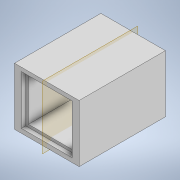
# Autodesk Inventor part: Part2
Saved by Autodesk Inventor 2022.6 (Build 266554010, 554A)
## iProperties
Created: 2025-03-19
Part Number: Part2
Material: Generic
Document SubType Name: Modeling
Designer: khinm
Density: 1 g/cm^3
Appearance: Default
Author: khinm
Autodesk Inventor part; units mm, degrees
ref_plane "XZ Plane" through (0, 0, 0) normal (0, 1, 0) x (-1, 0, 0)
ref_plane "XY Plane" through (0, 0, 0) normal (0, 0, 1) x (1, 0, 0)
sketch "Sketch1" plane through (0, 0, 0) normal (0, 0, 1) x (1, 0, 0)
  line L0 (-9.4982, 16.8551) -> (9.4982, 16.8551)
  line L1 (9.4982, 16.8551) -> (9.4982, 0)
  line L2 (9.4982, 0) -> (-9.4982, 0)
  line L3 (-9.4982, 0) -> (-9.4982, 16.8551)
  point P0 (0, 0)
  point P1 (0, 0)
  dimension "d0" = 16.8551
  dimension "d1" = 18.9965
  constraints: 8 end point, 2 parallel, 1 coincident, 1 horizontal, 1 midpoint, 1 perpendicular
  measures "d0" distance of L0.end L1.end
  measures "d1" distance of L0.start L0.end
extrude "Extrusion1" add sketch "Sketch1" along normal mid plane 25.4
sketch "Sketch2" plane through (0, 0, 12.7) normal (0, 0, 1) x (1, 0, 0)
  line L0 (-6.666, 14.9209) -> (6.666, 14.9209)
  line L1 (6.666, 14.9209) -> (6.666, 2.0723)
  line L2 (6.666, 2.0723) -> (-6.666, 2.0723)
  line L3 (-6.666, 2.0723) -> (-6.666, 14.9209)
  line L4 (-9.4982, 0) -> (9.4982, 0) projected
  point P0 (0, 0)
  point P1 (0, 0)
  point P2 (0, 2.0723)
  dimension "d4" = 12.8485
  dimension "d5" = 13.3321
  constraints: 8 end point, 2 midpoint, 2 parallel, 1 horizontal, 1 perpendicular, 1 vertical alignment
  measures "d4" distance of L0.end L1.end
  measures "d5" distance of L0.start L0.end
extrude "Extrusion2" cut sketch "Sketch2" against normal blind 22.86
ref_plane "Work Plane1" through (0, 0, 0) normal (1, 0, 0) x (0, 1, 0)
sketch "Sketch3" plane through (0, 0, 0) normal (1, 0, 0) x (0, 1, 0)
  line L0 (14.9209, 12.7) -> (14.9209, -10.16) projected
  line L1 (16.8551, 12.7) -> (0, 12.7) projected
  line L2 (15.7291, 12.7) -> (15.7291, 11.4381)
  line L3 (15.7291, 11.4381) -> (14.9209, 11.4381)
  line L4 (14.9209, 11.4381) -> (14.9209, 12.7)
  line L5 (15.7291, 12.7) -> (14.9209, 12.7)
  point P0 (0, 0)
  dimension "d9" = 1.2619
  dimension "d10" = 0.8082
  constraints: 8 end point, 3 perpendicular, 2 point on line, 1 collinear
  measures "d9" distance of L2.start L2.end
  measures "d10" distance of L3.end L2.end
sketch3d "3D Sketch1"
  line L0 (-6.666, 14.9209, 12.7) -> (-6.666, 2.0723, 12.7)
  line L1 (-6.666, 2.0723, 12.7) -> (6.666, 2.0723, 12.7)
  line L2 (6.666, 2.0723, 12.7) -> (6.666, 14.9209, 12.7)
  line L3 (6.666, 14.9209, 12.7) -> (-6.666, 14.9209, 12.7)
sweep "Sweep1" cut profiles "Sketch3" path "3D Sketch1"
body "Solid1"
